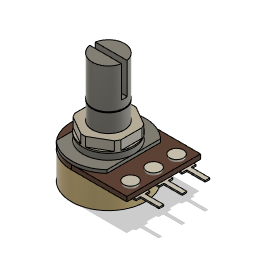
Potentiometer (Autodesk Fusion 360 design; units mm, degrees)
Autodesk Fusion 360 part; units mm, degrees
sketch "Sketch1" plane through (0, 0, 0) normal (0, 1, 0) x (1, 0, 0)
  circle A0 centre (0, 0) radius 8
  dimension "d1" = 16
  constraint coincident A0.centre origin
  measures "d1" diameter of A0
extrude "Extrude1" add sketch "Sketch1" along normal blind 6 makes body 1
sketch "Sketch3" plane through (0, 6, 0) normal (0, 1, 0) x (1, 0, 0)
  circle A0 centre (0, 0) radius 8
  line L0 (12, 8) -> (12, -8)
  line L1 (12, -8) -> (0, -8)
  line L2 (12, 8) -> (0, 8)
  circle A1 centre (0, 0) radius 8
  point P0 (-8, 0)
  point P1 (-8, 0)
  dimension "d7" = 20
  constraint vertical L0
  constraint coincident A0 L2.end
  constraint coincident A0 L1.end
  constraint tangent A0 L2
  constraint tangent A0 L1
  constraint perpendicular L0 L2
  constraint perpendicular L0 L1
  constraint coincident P1 P0
  measures "d7" distance of L0 P1
extrude "Extrude3" add sketch "Sketch3" along normal blind 1 separate body makes body 2
sketch "Sketch4" plane through (0, 7, 0) normal (0, 1, 0) x (-1, 0, 0)
  line L0 (-12, 8) -> (-12, -8)
  line L1 (-12, -8) -> (0, -8)
  arc A0 (0, -8) -> (0, 8) centre (0, 0) ccw
  line L2 (0, 8) -> (-12, 8)
  circle A1 centre (-9.8, 0) radius 1.5
  line L3 (-12, 8) -> (-12, -8)
  circle A2 centre (0, 0) radius 8
  line L4 (-12, 8) -> (-12, -8)
  line L5 (-12, -8) -> (0, -8)
  arc A3 (0, -8) -> (0, 8) centre (0, 0) ccw
  line L6 (0, 8) -> (-12, 8)
  dimension "d10" = 3
  dimension "d11" = 2.2
  constraint horizontal A0.centre A1.centre
  measures "d10" diameter of A1
  measures "d11" distance of A1.centre L3
extrude "Extrude4" add sketch "Sketch4" along normal blind 0.4 and the other way blind 1.3 separate body contours A1 makes body 3
sketch "Sketch5" plane through (0, 5.7, 0) normal (0, -1, 0) x (1, 0, 0)
  circle A0 centre (9.8, 0) radius 1.5
  line L0 (9.8, 1.5) -> (12.5, 1.5)
  line L1 (12.5, -1.5) -> (9.8, -1.5)
  line L2 (12, -8) -> (12, 8)
  line L3 (16.5, 0.5) -> (12.5, 0.5)
  line L4 (12.5, -0.5) -> (16.5, -0.5)
  line L5 (16.5, -0.5) -> (16.5, 0.5)
  line L6 (16.5, 0.5) -> (12.5, -0.5) construction
  line L7 (12.5, 0.5) -> (16.5, -0.5) construction
  line L8 (12.5, 1.5) -> (12.5, 0.5)
  line L9 (12.5, -0.5) -> (12.5, -1.5)
  line L10 (12.5, 0.5) -> (12.5, -0.5) construction
  point P0 (8.3, 0)
  point P1 (14.5, 0)
  dimension "d17" = 0.5
  dimension "d18" = 1
  dimension "d19" = 4
  constraint coincident A0 P0
  constraint horizontal A0.centre P0
  constraint coincident A0 L0.start
  constraint tangent A0 L0
  constraint perpendicular L0 L8
  constraint coincident A0 L1.end
  constraint tangent A0 L1
  constraint perpendicular L1 L8
  constraint horizontal L0
  constraint parallel L3 L4
  constraint horizontal L3
  constraint coincident L6 P1
  constraint coincident L7 P1
  constraint horizontal A0.centre P1
  constraint coincident L4.start L8
  constraint perpendicular L3 L5
  constraint vertical L9
  measures "d17" distance of L2.end L8
  measures "d18" distance of L3.start L4.end
  measures "d19" distance of L4.start L4.end
extrude "Extrude5" add sketch "Sketch5" against normal blind 0.3 separate body contours A0 L0 L1 L2 | L0 L1 L2 L3 L4 L5 L8 L9 makes body 4
combine "Combine1" operation add target body 3 tool bodies 4
pattern_linear "R-Pattern1" count 3 spacing 5 along (0, 0, 1) both ways of bodies 3 makes body 5 at (10.7, 5.7, -5.1667) makes body 6 at (10.7, 5.7, 5.1667)
sketch "Sketch6" plane through (0, 7, 0) normal (0, 1, 0) x (-1, 0, 0)
  circle A0 centre (0, 0) radius 8
  line L0 (5.5, -5.8095) -> (5.5, 5.8095)
  line L1 (-5.5, 5.8095) -> (-5.5, -5.8095)
  line L2 (5.5, 0) -> (-5.5, 0) construction
  line L3 (-12, 8) -> (-12, -8)
  line L4 (-12, -8) -> (0, -8)
  arc A1 (0, -8) -> (0, 8) centre (0, 0) ccw
  line L5 (0, 8) -> (-12, 8)
  dimension "d26" = 11
  constraint coincident A0 L0.start
  constraint coincident A0 L0.end
  constraint coincident A0 L1.start
  constraint coincident A0 L1.end
  constraint vertical L0
  constraint vertical L1
  constraint midpoint L0 L2.start
  constraint midpoint L1 L2.end
  constraint midpoint A0.centre L2
  measures "d26" distance of L0.start L1.end
extrude "Extrude6" add sketch "Sketch6" along normal blind 0.7 separate body contours A0 L0 L1 A1 makes body 7
sketch "Sketch7" plane through (0, 7.7, 0) normal (0, 1, 0) x (-1, 0, 0)
  line L0 (-5.5, 5.8095) -> (-5.5, -5.8095)
  arc A0 (-5.5, -5.8095) -> (5.5, -5.8095) centre (0, 0) ccw
  line L1 (5.5, -5.8095) -> (5.5, 5.8095)
  arc A1 (5.5, 5.8095) -> (-5.5, 5.8095) centre (0, 0) ccw
  circle A2 centre (0, 0) radius 5.5
  constraint concentric A0 A2
  constraint tangent L1 A2
extrude "Extrude7" add sketch "Sketch7" along normal blind 1.3 contours A2 bodies 7
sketch "Sketch8" plane through (0, 9, 0) normal (0, 1, 0) x (-1, 0, 0)
  circle A0 centre (0, 0) radius 5.5
  circle A1 centre (0, 0) radius 3.5
  dimension "d31" = 7
  constraint concentric A0 A1
  measures "d31" diameter of A1
extrude "Extrude8" add sketch "Sketch8" along normal blind 6.3 contours A1 bodies 7
sketch "Sketch1 (2)" plane through (0, 15.3, 0) normal (0, 1, 0) x (-1, 0, 0) in component "Rotary top"
  circle A0 centre (0, 0) radius 3.5
extrude "Extrude1'" add sketch "Sketch1 (2)" along normal blind 8.7 separate body makes body 8 in component "Rotary top"
chamfer "Chamfer1" distance 0.1 angle 45 1 edges at (3.2631, 15.3, -1.2657) on bodies 8 in component "Rotary top"
chamfer "Chamfer1'" distance 0.1 angle 45 1 edges at (3.2631, 15.3, -1.2657) on bodies 7
sketch "Sketch2" plane through (0, 24, 0) normal (0, 1, 0) x (-1, 0, 0) in component "Rotary top"
  circle A0 centre (0, 0) radius 3.5
  line L0 (3.4482, -0.6) -> (-3.4482, -0.6)
  line L1 (3.4482, 0.6) -> (-3.4482, 0.6)
  line L2 (0, -0.6) -> (0, 0.6) construction
  dimension "d38" = 1.2
  constraint coincident A0 L0.start
  constraint coincident A0 L0.end
  constraint coincident A0 L1.start
  constraint coincident A0 L1.end
  constraint midpoint L0 L2.start
  constraint midpoint L1 L2.end
  constraint horizontal L0
  constraint horizontal L1
  constraint midpoint A0.centre L2
  measures "d38" distance of L0 L1
extrude "Extrude2" cut sketch "Sketch2" against normal blind 6.8 contours A0 L0 L1 bodies 8 in component "Rotary top"
sketch "Sketch1 (3)" plane through (0, 9, 0) normal (0, 1, 0) x (-1, 0, 0) in component "Nut and washer"
  circle A0 centre (0, 0) radius 3.5
  circle A1 centre (0, 0) radius 5.5
  circle A2 centre (0, 0) radius 3.5
  circle A3 centre (0, 0) radius 5.75
  dimension "d53" = 11.5
  constraint coincident A0.centre A1.centre
  measures "d53" diameter of A3
extrude "Extrude1''" add sketch "Sketch1 (3)" along normal blind 0.3 separate body contours A1 makes body 9 in component "Nut and washer"
sketch "Sketch2 (2)" plane through (0, 9.3, 0) normal (0, 1, 0) x (-1, 0, 0) in component "Nut and washer"
  circle A0 centre (0, 0) radius 3.5
  circle A1 centre (0, 0) radius 5.5
  line L0 (-5, -2.8868) -> (0, -5.7735)
  line L1 (0, -5.7735) -> (5, -2.8868)
  line L2 (5, -2.8868) -> (5, 2.8868)
  line L3 (5, 2.8868) -> (0, 5.7735)
  line L4 (0, 5.7735) -> (-5, 2.8868)
  line L5 (-5, 2.8868) -> (-5, -2.8868)
  dimension "d56" = 10
  constraint coincident A0.centre A1.centre
  constraint vertical L5
  measures "d56" distance of L2 L5
extrude "Extrude2'" add sketch "Sketch2 (2)" along normal blind 2 contours A1 L0 L1 L2 L3 L4 L5 bodies 9 in component "Nut and washer"
component "Rotary top" placed x (1, 0, 0) y (0, 1, 0) z (0, 0, 1) at (0, 0, 0)
component "Nut and washer" placed x (1, 0, 0) y (0, 1, 0) z (0, 0, 1) at (0, 0, 0)
